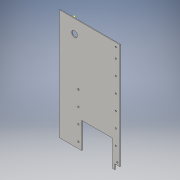
# Autodesk Inventor part: GearboxPlateRev3
Saved by Autodesk Inventor 2016 (Build 200138000, 138)
## iProperties
Created: 2017-01-27
Part Number: GearboxPlateRev3
Material: Generic
Document SubType Name: Modeling
Designer: madsenn
Density: 1 g/cm^3
Appearance: Default
Author: madsenn
Autodesk Inventor part; units mm, degrees
ref_plane "YZ Plane" through (0, 0, 0) normal (1, 0, 0) x (0, 1, 0)
ref_plane "XZ Plane" through (0, 0, 0) normal (0, 1, 0) x (-1, 0, 0)
ref_plane "XY Plane" through (0, 0, 0) normal (0, 0, 1) x (1, 0, 0)
sketch "Sketch1" plane through (0, 0, 0) normal (0, 0, 1) x (1, 0, 0)
  line L0 (229.6952, -414.7737) -> (228.902, -414.7737)
  line L1 (204.202, -567.6898) -> (204.202, -542.0358)
  line L2 (204.202, -542.0358) -> (229.856, -542.0358)
  line L3 (204.202, -567.6898) -> (-74.944, -567.6898)
  line L4 (-74.944, -567.6898) -> (-74.944, -265.633)
  line L5 (229.856, -542.0358) -> (229.856, -8.8898)
  line L6 (229.856, -8.8898) -> (188.7123, -8.8898)
  circle A0 centre (20.5783, -308.8638) radius 3.5687
  circle A1 centre (20.574, -385.0638) radius 3.5687
  circle A2 centre (20.574, -461.2638) radius 3.5687
  circle A3 centre (20.574, -537.4638) radius 3.5687
  circle A4 centre (217.156, -529.3358) radius 3.5687
  circle A5 centre (209.282, -461.2638) radius 3.5687
  circle A6 centre (209.282, -385.0638) radius 3.5687
  circle A7 centre (209.282, -308.8638) radius 3.5687
  circle A8 centre (209.282, -232.6638) radius 3.5687
  circle A9 centre (209.2863, -156.4638) radius 3.5687
  circle A10 centre (209.282, -80.2638) radius 3.5687
  circle A11 centre (209.282, -29.4638) radius 3.5687
  line L7 (229.856, -8.8898) -> (-74.944, -8.8898)
  line L8 (-74.944, -8.8898) -> (-74.944, -567.6898)
  line L9 (191.756, -567.6898) -> (37.6288, -567.6898)
  line L10 (37.6288, -567.6898) -> (37.6288, -435.6098)
  line L11 (37.6288, -435.6098) -> (191.756, -435.6098)
  line L12 (191.756, -435.6098) -> (191.756, -567.6898)
  circle A12 centre (1.256, -76.1998) radius 189.4332 construction
  circle A13 centre (1.256, -76.1998) radius 14.2875
  point P0 (0, 0)
  dimension "d0" = 25.654
  dimension "d3" = 558.8
  dimension "d5" = 76.2
  dimension "d6" = 20.5697
  dimension "d7" = 20.574
  dimension "d9" = 76.2
  dimension "d10" = 76.2
  dimension "d11" = 76.2
  dimension "d12" = 76.2
  dimension "d13" = 25.654
  dimension "d14" = 12.7
  dimension "d15" = 76.2
  dimension "d16" = 76.2
  dimension "d17" = 76.2
  dimension "d18" = 43.2308
  dimension "d23" = 7.1374
  dimension "d24" = 7.1374
  dimension "d25" = 7.1374
  dimension "d26" = 7.1374
  dimension "d27" = 7.1374
  dimension "d28" = 7.1374
  dimension "d29" = 7.1374
  dimension "d30" = 7.1374
  dimension "d31" = 7.1374
  dimension "d32" = 7.1374
  dimension "d33" = 7.1374
  dimension "d34" = 7.1374
  dimension "d35" = 304.8
  dimension "d36" = 12.7
  dimension "d37" = 106.426
  dimension "d38" = 188.7037
  dimension "d39" = 188.708
  dimension "d40" = 188.708
  dimension "d41" = 188.708
  dimension "d42" = 20.574
  dimension "d43" = 20.574
  dimension "d44" = 20.574
  dimension "d45" = 30.226
  dimension "d46" = 20.574
  dimension "d47" = 12.446
  dimension "d48" = 154.1272
  dimension "d49" = 132.08
  dimension "d50" = 378.8664
  dimension "d51" = 76.2
  dimension "d56" = 491.49
  dimension "d57" = 28.575
  dimension "d61" = 50.8
  constraints: 26 end point, 14 centre point, 13 coincident, 4 horizontal, 4 perpendicular, 3 parallel, 1 collinear, 1 point on line, 1 vertical, 1 vertical alignment
  measures "d0" distance of L2.end L1.end
  measures "d3" distance between parallel lines of L3 L6
  measures "d5" distance of point (209.286, -156.464) point (209.282, -80.264)
  measures "d6" distance from line of L5 point (209.286, -156.464)
  measures "d7" distance from line of L5 point (209.282, -232.664)
  measures "d9" distance of point (209.282, -232.664) point (209.286, -156.464)
  measures "d10" distance of point (209.282, -232.664) point (209.282, -308.864)
  measures "d11" distance of point (209.282, -385.064) point (209.282, -308.864)
  measures "d12" distance of point (209.282, -461.264) point (209.282, -385.064)
  measures "d13" distance between parallel lines of L3 L2
  measures "d14" distance from line of L2 point (217.156, -529.336)
  measures "d15" distance of point (20.574, -385.064) point (20.578, -308.864)
  measures "d16" distance of point (20.574, -461.264) point (20.574, -385.064)
  measures "d17" distance of point (20.574, -537.464) point (20.574, -461.264)
  measures "d18" vertical distance of L4.end point (20.578, -308.864)
  measures "d23" diameter of A0
  measures "d24" diameter of A1
  measures "d25" diameter of A2
  measures "d26" diameter of A3
  measures "d27" diameter of A4
  measures "d28" diameter of A5
  measures "d29" diameter of A6
  measures "d30" diameter of A7
  measures "d31" diameter of A8
  measures "d32" diameter of A9
  measures "d33" diameter of A10
  measures "d34" diameter of A11
  measures "d35" distance between parallel lines of L5 L8
  measures "d36" distance from line of L5 A4.centre
  measures "d37" distance from line of L3 point (209.282, -461.264)
  measures "d38" horizontal distance of point (209.282, -232.664) point (20.578, -308.864)
  measures "d39" horizontal distance of point (209.282, -308.864) point (20.574, -385.064)
  measures "d40" horizontal distance of point (209.282, -385.064) point (20.574, -461.264)
  measures "d41" horizontal distance of point (209.282, -461.264) point (20.574, -537.464)
  measures "d42" distance from line of L5 point (209.282, -308.864)
  measures "d43" distance from line of L5 point (209.282, -385.064)
  measures "d44" distance from line of L5 point (209.282, -461.264)
  measures "d45" distance from line of L3 point (20.574, -537.464)
  measures "d46" distance from line of L5 point (209.282, -80.264)
  measures "d47" distance between parallel lines of L1 L12
  measures "d48" distance between parallel lines of L12 L10
  measures "d49" distance between parallel lines of L3 L11
  measures "d50" diameter of A12
  measures "d51" distance from line of L8 A12.centre
  measures "d56" distance from line of L3 A12.centre
  measures "d57" diameter of A13
  measures "d61" distance of point (209.282, -80.264) point (209.282, -29.464)
extrude "Extrusion1" add sketch "Sketch1" along normal blind 3.175 contours L3 L12 L11 L10 L4 L8 L7 L6 L5 L2 L1
sketch "Sketch2" plane through (0, 0, 3.175) normal (0, 0, 1) x (1, 0, 0)
  point P0 (0, 0)
body "Solid1"
